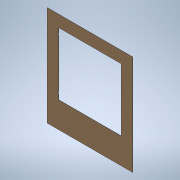
# Autodesk Inventor part: frente
Saved by Autodesk Inventor 2022 (Build 260153000, 153)
## iProperties
Created: 2022-02-18
Part Number: frente
Material: MDF - Chapa de fibra de média densidade
Document SubType Name: Modeling
Designer: mathe
Density: 0.8 g/cm^3
Appearance: Papelão - Corrugado
Author: mathe
Autodesk Inventor part; units mm, degrees
ref_plane "YZ Plane" through (0, 0, 0) normal (1, 0, 0) x (0, 1, 0)
ref_plane "XZ Plane" through (0, 0, 0) normal (0, 1, 0) x (-1, 0, 0)
ref_plane "XY Plane" through (0, 0, 0) normal (0, 0, 1) x (1, 0, 0)
sketch "Esboço1" plane through (0, 0, 0) normal (0, 0, 1) x (1, 0, 0)
  line L0 (0, 0) -> (600, 0)
  line L1 (600, 0) -> (600, 700)
  line L2 (600, 700) -> (0, 700)
  line L3 (0, 700) -> (0, 0)
  dimension "d0" = 600
  dimension "d1" = 700
  constraints: 8 end point, 2 parallel, 1 horizontal, 1 perpendicular
  measures "d0" distance of L2.end L1.end
  measures "d1" distance of L1.end L0.end
extrude "Extrusão1" add sketch "Esboço1" along normal blind 3
sketch "Esboço2" plane through (0, 0, 3) normal (0, 0, 1) x (1, 0, 0)
  line L0 (80, 620) -> (520, 620)
  line L1 (520, 620) -> (520, 180)
  line L2 (520, 180) -> (80, 180)
  line L3 (80, 180) -> (80, 620)
  line L4 (0, 700) -> (0, 0) projected
  line L5 (600, 0) -> (600, 700) projected
  line L6 (600, 700) -> (0, 700) projected
  line L7 (0, 0) -> (600, 0) projected
  dimension "d4" = 80
  dimension "d5" = 80
  dimension "d6" = 80
  dimension "d7" = 180
  constraints: 8 end point, 2 parallel, 1 horizontal, 1 perpendicular
  measures "d4" distance between parallel lines of L4 L3
  measures "d5" distance between parallel lines of L5 L1
  measures "d6" distance between parallel lines of L6 L0
  measures "d7" distance between parallel lines of L7 L2
extrude "Extrusão2" cut sketch "Esboço2" against normal blind 10 contours L0 L1 L2 L3
fillet "Arredondamento1" radius 2 4 edges at (80, 620, 1.5) (520, 620, 1.5) (520, 180, 1.5) (80, 180, 1.5)
sketch "Esboço3" plane through (0, 0, 0) normal (0, 0, -1) x (-1, 0, 0)
  point P0 (0, 0)
  point P1 (-75, 220)
  point P2 (-75, 227)
  point P3 (-75, 580)
  point P4 (-75, 573)
hole "Furo1" at (75, 220, 0) at (75, 227, 0) at (75, 580, 0) at (75, 573, 0) direction (0, 0, 1) diameter 2 end through all
sketch "Esboço4" plane through (0, 0, 0) normal (0, 0, -1) x (-1, 0, 0)
  line L0 (-80, 618) -> (-80, 182) projected
  line L1 (-80, 232.8077) -> (-77, 232.8077)
  line L2 (-77, 232.8077) -> (-77, 214.8077)
  line L3 (-77, 214.8077) -> (-80, 214.8077)
  line L4 (-80, 214.8077) -> (-80, 232.8077)
  line L5 (-80, 586.0371) -> (-77, 586.0371)
  line L6 (-77, 586.0371) -> (-77, 568.0371)
  line L7 (-77, 568.0371) -> (-80, 568.0371)
  line L8 (-80, 568.0371) -> (-80, 586.0371)
  point P0 (0, 0)
  point P1 (-80, 586.0371)
  dimension "d19" = 3
  dimension "d20" = 18
  dimension "d21" = 3
  dimension "d22" = 18
  constraints: 16 end point, 4 parallel, 2 horizontal, 2 perpendicular
  measures "d19" distance between parallel lines of L4 L2
  measures "d20" distance between parallel lines of L3 L1
  measures "d21" distance between parallel lines of L8 L6
  measures "d22" distance between parallel lines of L7 L5
extrude "Extrusão3" cut sketch "Esboço4" against normal blind 10
